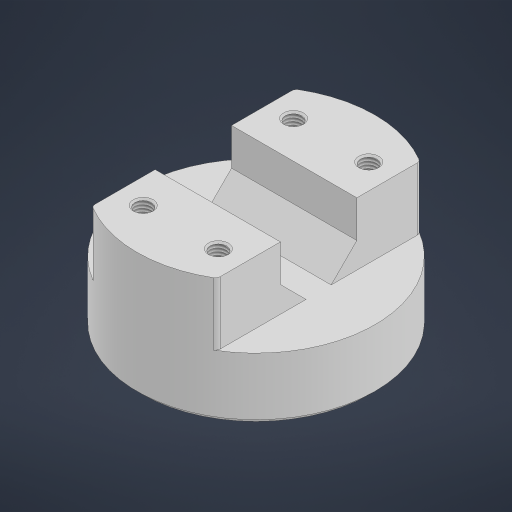
# Autodesk Inventor part: HM1_FIXT2-001
Saved by Autodesk Inventor 2024.3 (Build 283343000, 343)
## iProperties
Created: 2024-10-19
Part Number: HM1_FIXT2-001
Material: Generic
Document SubType Name: Modeling
Designer: fablabadmin
Density: 1 g/cm^3
Appearance: Default
Author: fablabadmin
Autodesk Inventor part; units mm, degrees
ref_plane "YZ Plane" through (0, 0, 0) normal (1, 0, 0) x (0, 1, 0)
ref_plane "XZ Plane" through (0, 0, 0) normal (0, 1, 0) x (-1, 0, 0)
ref_plane "XY Plane" through (0, 0, 0) normal (0, 0, 1) x (1, 0, 0)
sketch "Sketch1" plane through (0, 0, 0) normal (0, 1, 0) x (-1, 0, 0)
  circle A0 centre (0, 0) radius 47.5
  dimension "d0" = 95
  constraints: 1 centre point, 1 coincident
  measures "d0" diameter of A0
extrude "Extrusion1" add sketch "Sketch1" along normal mid plane 50
sketch "Sketch4" plane through (0, 0, 0) normal (1, 0, 0) x (0, 1, 0)
  line L0 (-25, 47.5) -> (-25, -47.5) projected
  line L1 (25, -47.5) -> (25, 47.5) projected
  line L2 (-42, 0) -> (42, 0) projected
  line L3 (25, 15.25) -> (10.25, 15.25)
  line L4 (10.25, 15.25) -> (0, 5)
  line L5 (0, 5) -> (0, 0)
  line L6 (25, -15.25) -> (10.25, -15.25)
  line L7 (10.25, -15.25) -> (0, -5)
  line L8 (0, -5) -> (0, 0)
  dimension "d22" = 30.5
  dimension "d23" = 45
  dimension "d24" = 10
  dimension "d25" = 25
  constraints: 12 end point, 3 symmetric about line, 2 perpendicular, 1 midpoint, 1 point on line
  measures "d22" diameter of L3 L2
  measures "d23" angle of L5 L4
  measures "d24" diameter of L4.end L2
  measures "d25" distance from line of L1 L4.end
extrude "Extrusion3" cut sketch "Sketch4" along normal through all both and the other way through all
sketch "Sketch5" plane through (0, 25, 0) normal (0, 1, 0) x (1, 0, 0)
  line L0 (-66.5, 0) -> (66.5, 0) construction
  line L1 (0, 66.5) -> (0, -66.5) construction
  arc A0 (44.9854, 15.25) -> (-44.9854, 15.25) centre (0, 0) ccw construction
  line L2 (-47.5, 40.3887) -> (-25, 40.3887)
  line L3 (-25, 40.3887) -> (-25, -40.3887)
  line L4 (-25, -40.3887) -> (-47.5, -40.3887)
  line L5 (-47.5, -40.3887) -> (-47.5, 40.3887)
  arc A1 (-47.2361, 5) -> (-47.2361, -5) centre (0, 0) ccw projected
  line L6 (47.5, 40.3887) -> (25, 40.3887)
  line L7 (25, 40.3887) -> (25, -40.3887)
  line L8 (25, -40.3887) -> (47.5, -40.3887)
  line L9 (47.5, -40.3887) -> (47.5, 40.3887)
  arc A2 (47.2361, -5) -> (47.2361, 5) centre (0, 0) ccw
  dimension "d28" = 50
  constraints: 16 end point, 6 symmetric about line, 3 point on circle, 2 parallel, 1 centre point, 1 horizontal, 1 perpendicular, 1 tangent, 2 other
  measures "d28" distance between parallel lines of L7 L3
extrude "Extrusion4" cut sketch "Sketch5" against normal up to surface (25 mm away)
sketch "Sketch6" plane through (0, 25, 0) normal (0, 1, 0) x (1, 0, 0)
  line L0 (15, -30) -> (-15, -30) construction
  line L1 (-15, -30) -> (-15, 30) construction
  line L2 (-15, 30) -> (15, 30) construction
  line L3 (15, 30) -> (15, -30) construction
  line L4 (15, -30) -> (-15, 30) construction
  line L5 (-15, -30) -> (15, 30) construction
  point P0 (0, 0)
  dimension "d31" = 30
  dimension "d32" = 60
  constraints: 12 end point, 4 coincident, 2 midpoint, 2 parallel, 1 horizontal, 1 perpendicular
  measures "d31" distance of L1.end L2.end
  measures "d32" distance of L0.end L1.end
hole "Hole2" at (-15, 25, -30) at (15, 25, -30) at (-15, 25, 30) at (15, 25, 30) direction (0, -1, 0) diameter 6.647 depth 20.4 tip angle 118 countersink diameter 8 countersink angle 90 thread size "M8x1.25" class "6H" standard "ISO Metric profile"
fillet "Fillet1" radius 2 4 edges at (-25, 12.5, -40.3887) (-25, 12.5, 40.3887) (25, 12.5, -40.3887) (25, 12.5, 40.3887)
chamfer "Chamfer3" distance 2 angle 45 1 edges at (47.5, -25, 0)
sketch "Sketch7" plane through (0, -25, 0) normal (0, -1, 0) x (1, 0, 0)
  circle A0 centre (0, 0) radius 15 construction
  circle A1 centre (0, 0) radius 19 construction
  dimension "d44" = 4
  dimension "d45" = 30
  constraints: 2 centre point, 2 coincident, 2 other
  measures "d44" radial gap between concentric circles of A0 A1
  measures "d45" diameter of A0
mark "Mark1"
body "Solid1"
